Autodesk Fusion 360 part; units mm, degrees
(part 5 of 5)
sketch "Sketch1" plane through (0, 0, 0) normal (0, 0, 1) x (1, 0, 0)
  circle A0 centre (0, 0) radius 1.5
  line L0 (0, 0) -> (29.5, 0) construction
  circle A1 centre (29.5, 0) radius 1.5
  arc A2 (11.3878, -17.4724) -> (12.4, -15.6206) centre (10.2, -15.6206) ccw construction
  line L1 (3, -19.6) -> (3, -7.6) construction
  arc A3 (18.1137, -9.9501) -> (17.1, -11.8029) centre (19.3, -11.8029) ccw construction
  line L2 (29.5, 5) -> (28.4595, 5)
  line L3 (11.9527, 9.1208) -> (3.8379, 5.5832)
  arc A4 (1.2, -13.6) -> (-0.8, -13.6) centre (0.2, -13.6) ccw construction
  arc A5 (13.4019, -3.7339) -> (16.0981, -3.7339) centre (14.75, -1.6285) ccw construction
  arc A6 (33.75, -2.6339) -> (29.5, 5) centre (29.5, 0) ccw
  circle A7 centre (0, 0) radius 1.5
  line L4 (12.4, -11.8029) -> (12.4, -15.6206) construction
  arc A8 (7.2, -16.1338) -> (10.5878, -17.9855) centre (9.4, -16.1338) ccw construction
  arc A9 (17.5473, 9.1208) -> (11.9527, 9.1208) centre (14.75, 2.704) ccw
  line L5 (7.2, -16.1338) -> (7.2, -9.4629) construction
  line L6 (9.0471, -8.4523) -> (11.3863, -9.9501) construction
  arc A10 (-3.8, -4.2143) -> (-4.25, -2.6339) centre (-6.8, -4.2143) ccw construction
  arc A11 (9.3018, 1.2017) -> (9.1273, -0.9969) centre (9.8014, 0.0558) ccw construction
  line L7 (25.6621, 5.5832) -> (17.5473, 9.1208)
  line L8 (1.0405, 5) -> (0, 5)
  line L9 (15.0697, 3.4373) -> (20.1982, 1.2017) construction
  arc A12 (22.3, -9.4629) -> (20.4529, -8.4523) centre (21.1, -9.4629) ccw construction
  arc A13 (1.0405, 5) -> (3.8379, 5.5832) centre (1.0405, 12) ccw
  line L10 (17.1, -15.6206) -> (17.1, -11.8029) construction
  line L11 (9.3018, 1.2017) -> (14.4303, 3.4373) construction
  circle A14 centre (29.5, 0) radius 1.5
  arc A15 (33.75, -2.6339) -> (33.3, -4.2143) centre (36.3, -4.2143) ccw construction
  arc A16 (20.3727, -0.9969) -> (20.1982, 1.2017) centre (19.6986, 0.0558) ccw construction
  arc A17 (0, 5) -> (-4.25, -2.6339) centre (0, 0) ccw
  line L12 (18.9122, -17.9855) -> (18.1122, -17.4724) construction
  line L13 (5, -7.6) -> (5, -19.6) construction
  arc A18 (15.0697, 3.4373) -> (14.4303, 3.4373) centre (14.75, 2.704) ccw construction
  line L14 (11.3878, -17.4724) -> (10.5878, -17.9855) construction
  line L15 (18.1137, -9.9501) -> (20.4529, -8.4523) construction
  arc A19 (12.4, -11.8029) -> (11.3863, -9.9501) centre (10.2, -11.8029) ccw construction
  arc A20 (5, -7.6) -> (3, -7.6) centre (4, -7.6) ccw construction
  line L16 (24.5, -19.6) -> (24.5, -7.6) construction
  arc A21 (25.6621, 5.5832) -> (28.4595, 5) centre (28.4595, 12) ccw
  line L17 (20.3727, -0.9969) -> (16.0981, -3.7339) construction
  arc A22 (3, -19.6) -> (5, -19.6) centre (4, -19.6) ccw construction
  arc A23 (18.9122, -17.9855) -> (22.3, -16.1338) centre (20.1, -16.1338) ccw construction
  arc A24 (17.1, -15.6206) -> (18.1122, -17.4724) centre (19.3, -15.6206) ccw construction
  line L18 (13.4019, -3.7339) -> (9.1273, -0.9969) construction
  arc A25 (9.0471, -8.4523) -> (7.2, -9.4629) centre (8.4, -9.4629) ccw construction
  line L19 (26.5, -7.6) -> (26.5, -19.6) construction
  arc A26 (26.5, -7.6) -> (24.5, -7.6) centre (25.5, -7.6) ccw construction
  line L20 (22.3, -9.4629) -> (22.3, -16.1338) construction
  arc A27 (30.3, -13.6) -> (28.3, -13.6) centre (29.3, -13.6) ccw construction
  circle A28 centre (0, 0) radius 5
  circle A29 centre (29.5, 0) radius 5
  line L21 (23.2644, 0.0831) -> (15.1496, 3.6207)
  arc A30 (15.1496, 3.6207) -> (14.3504, 3.6207) centre (14.75, 2.704) ccw
  line L22 (14.3504, 3.6207) -> (6.2356, 0.0831)
  line L23 (6.2356, 0.0831) -> (4.9783, -0.4649)
  line L24 (23.2644, 0.0831) -> (24.5217, -0.4649)
  point P0 (14.75, -5.1)
  dimension "d35" = 3
  dimension "d36" = 29.5
  dimension "d37" = 3
  dimension "d38" = -6
  constraint coincident A0.centre L0.start
  constraint horizontal L0
  constraint coincident L0.end A1.centre
  constraint concentric A7 A28
  constraint coincident A10.end A28
  constraint coincident A6.start A29
  constraint tangent A15 A29
  constraint coincident A28 L23.end
  constraint collinear L22 L23
  constraint coincident A29 L24.end
  constraint collinear L21 L24
  measures "d35" diameter of A0
  measures "d36" distance of A0.centre L0.end
  measures "d37" diameter of A1
extrude "Extrude3" add sketch "Sketch1" along normal blind 2
fillet "Fillet3" radius 3 2 edges at (4.9783, -0.4649, 1) (24.5217, -0.4649, 1)

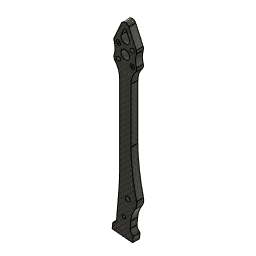
design "arm_front_6mm"
Autodesk Fusion 360 part; units mm, degrees
sketch "Sketch1" plane through (0, 0, 0) normal (0, 0, 1) x (1, 0, 0)
  circle A0 centre (0, 0) radius 3.8
  dimension "d2" = 7.6
  constraint coincident A0.centre origin
  measures "d2" diameter of A0
sketch "Sketch2" plane through (0, 0, 0) normal (0, 0, 1) x (1, 0, 0)
  arc A0 (28.2898, -146.7842) -> (30.0064, -147.0869) centre (30.8779, -137.1249) ccw construction
  arc A1 (9.3424, -112.1265) -> (12.7274, -116.0513) centre (22.2229, -104.4394) ccw construction
  line L0 (9.8518, -167.6702) -> (17.4021, -163.8233) construction
  circle A2 centre (2.1789, -108.5649) radius 3.375 construction
  line L1 (100.4519, -39.9064) -> (12.7274, -116.0513) construction
  line L2 (28.2898, -146.7842) -> (23.615, -145.5316) construction
  arc A3 (30.9564, -136.2283) -> (29.2133, -136.2283) centre (30.0848, -146.1903) ccw construction
  arc A4 (2.3786, -152.7505) -> (5.279, -154.7068) centre (4.371, -152.9248) ccw construction
  arc A5 (100.4519, -39.9064) -> (105.7604, -37.9868) centre (99.4908, -28.9484) ccw construction
  line L3 (18.4399, -134.3914) -> (17.361, -146.7224) construction
  line L4 (22.8776, -144.4785) -> (23.4829, -137.5592) construction
  arc A6 (-11.1082, -168.6356) -> (3.7484, -173.4033) centre (-3.1387, -169.3329) ccw construction
  arc A7 (23.3547, -162.6662) -> (17.4021, -163.8233) centre (22.396, -173.6243) ccw construction
  line L5 (-5.7907, -107.8678) -> (-7.6374, -128.9799)
  arc A8 (-9.2616, -147.5287) -> (-11.8245, -142.975) centre (-13.8718, -147.1253) ccw construction
  line L6 (4.7746, -145.5276) -> (6.1209, -144.398) construction
  line L7 (24.392, -136.6501) -> (29.2133, -136.2283) construction
  arc A9 (-10.9528, -133.0126) -> (-7.6374, -128.9799) centre (-12.2491, -128.5675) ccw
  circle A10 centre (27.1493, -126.0578) radius 1.5 construction
  line L8 (6.9668, -134.7286) -> (5.8373, -133.3824) construction
  line L9 (-9.2616, -147.5287) -> (-11.1082, -168.6356) construction
  arc A11 (22.8776, -144.4785) -> (23.615, -145.5316) centre (23.8738, -144.5656) ccw construction
  circle A12 centre (24.4911, -156.4418) radius 1.5 construction
  arc A13 (7.9279, -124.4303) -> (4.7319, -125.8533) centre (6.7243, -126.0276) ccw construction
  arc A14 (9.8518, -167.6702) -> (3.7484, -173.4033) centre (16.6616, -181.0354) ccw construction
  circle A15 centre (-3.7013, -153.9753) radius 1.5 construction
  arc A16 (9.3424, -112.1265) -> (-5.7907, -107.8678) centre (2.1789, -108.5649) ccw construction
  arc A17 (24.392, -136.6501) -> (23.4829, -137.5592) centre (24.4791, -137.6463) ccw construction
  line L10 (15.7692, -149.4168) -> (5.279, -154.7068) construction
  line L11 (2.3786, -152.7505) -> (2.6542, -149.601) construction
  circle A18 centre (31.9218, -131.7454) radius 1.5 construction
  line L12 (7.9279, -124.4303) -> (17.3401, -131.4615) construction
  circle A19 centre (-3.1387, -169.3329) radius 3.375 construction
  line L13 (4.4564, -129.0028) -> (4.7319, -125.8533) construction
  arc A20 (4.4564, -129.0028) -> (5.8373, -133.3824) centre (10.4336, -129.5257) ccw construction
  circle A21 centre (-1.043, -123.5913) radius 1.5
  spline S0 degree 5 poles (17.3401, -131.4615) (17.4524, -131.5454) (17.6596, -131.7229) (17.9183, -132.0182) (18.171, -132.4622) (18.3701, -133.0729) (18.4504, -133.5889) (18.4644, -133.9863) (18.4517, -134.2556) (18.4399, -134.3914) knots 0 0 0 0 0 0 0.2 0.4 0.6 0.8 1 1 1 1 1 1 construction
  circle A22 centre (30.1786, -151.6693) radius 1.5 construction
  spline S1 degree 5 poles (17.361, -146.7224) (17.3492, -146.8581) (17.3149, -147.1256) (17.232, -147.5145) (17.0634, -148.0088) (16.7613, -148.5756) (16.4353, -148.9689) (16.1293, -149.2149) (15.8944, -149.3537) (15.7692, -149.4168) knots -1 -1 -1 -1 -1 -1 -0.8 -0.6 -0.4 -0.2 0 0 0 0 0 0 construction
  arc A23 (4.7746, -145.5276) -> (2.6542, -149.601) centre (8.6313, -150.1239) ccw construction
  line L14 (-10.9528, -133.0126) -> (-11.8245, -142.975)
  line L15 (6.1209, -144.398) -> (6.9668, -134.7286) construction
  circle A24 centre (2.1789, -108.5649) radius 2
  line L16 (0.1865, -108.3907) -> (-1.6602, -129.5027) construction
  arc A25 (4.317, -130.0255) -> (6.882, -134.5726) centre (8.9303, -130.4201) ccw
  line L17 (6.882, -134.5726) -> (6.0108, -144.535)
  line L18 (-11.3887, -137.9938) -> (6.5439, -139.5619)
  circle A26 centre (2.1789, -108.5649) radius 8
  line L19 (4.317, -130.0255) -> (4.8399, -124.0484)
  spline S2 degree 5 poles (4.8399, -124.0484) (4.8815, -123.5731) (4.9918, -122.6298) (5.2386, -121.2367) (5.7136, -119.4197) (6.5081, -117.2134) (7.2997, -115.51) (7.9954, -114.2779) (8.5094, -113.4794) (8.779, -113.0859) knots 0 0 0 0 0 0 0.2 0.4 0.6 0.8 1 1 1 1 1 1
  line L20 (0, 0) -> (13.2638, -13.2638) construction
  line L21 (0, 0) -> (18.7579, 0) construction
  line L22 (7.566, -5.4447) -> (6.7175, -4.5962)
  arc A27 (6.7175, -4.5962) -> (4.5962, -6.7175) centre (5.6569, -5.6569) ccw
  line L23 (4.5962, -6.7175) -> (5.4447, -7.566)
  arc A28 (5.4447, -7.566) -> (7.566, -5.4447) centre (6.5054, -6.5054) ccw
  line L24 (7.566, -7.566) -> (4.5962, -4.5962) construction
  arc A29 (4.5962, 6.7175) -> (6.7175, 4.5962) centre (5.6569, 5.6569) ccw
  line L25 (5.4447, 7.566) -> (4.5962, 6.7175)
  arc A30 (7.566, 5.4447) -> (5.4447, 7.566) centre (6.5054, 6.5054) ccw
  line L26 (6.7175, 4.5962) -> (7.566, 5.4447)
  arc A31 (-6.7175, 4.5962) -> (-4.5962, 6.7175) centre (-5.6569, 5.6569) ccw
  line L27 (-7.566, 5.4447) -> (-6.7175, 4.5962)
  arc A32 (-5.4447, 7.566) -> (-7.566, 5.4447) centre (-6.5054, 6.5054) ccw
  line L28 (-4.5962, 6.7175) -> (-5.4447, 7.566)
  arc A33 (-4.5962, -6.7175) -> (-6.7175, -4.5962) centre (-5.6569, -5.6569) ccw
  line L29 (-5.4447, -7.566) -> (-4.5962, -6.7175)
  arc A34 (-7.566, -5.4447) -> (-5.4447, -7.566) centre (-6.5054, -6.5054) ccw
  line L30 (-6.7175, -4.5962) -> (-7.566, -5.4447)
  line L31 (0, 0) -> (0, -132.816) construction
  line L32 (-5, -105.0346) -> (-5, -20)
  spline S3 degree 5 poles (-5.7907, -107.8678) (-5.7382, -107.2682) (-5.6366, -106.0687) (-5.4939, -104.2686) (-5.3227, -101.867) (-5.1465, -98.863) (-5.0482, -96.458) (-5.0088, -94.6529) (-5, -93.4489) (-5, -92.8467) knots 0 0 0 0 0 0 0.2 0.4 0.6 0.8 1 1 1 1 1 1
  line L33 (5, -101.0789) -> (5, -20)
  line L34 (0, 24.5) -> (0, 0) construction
  circle A35 centre (0, 21) radius 3.5
  circle A36 centre (-6.5054, 6.5054) radius 3.5
  circle A37 centre (-6.5054, -6.5054) radius 3.5
  line L35 (0, 0) -> (-9, 0) construction
  arc A38 (-9.8421, -5.4488) -> (-9.8421, 5.4488) centre (-27.0494, 0) ccw
  line L36 (-5, -20) -> (5, -20) construction
  arc A39 (-5, -20) -> (-9.1588, -8.7878) centre (-22.1936, -20) ccw
  line L37 (-9.6985, 7.9385) -> (-3.1931, 22.4331)
  line L38 (9.6985, 7.9385) -> (3.1931, 22.4331)
  circle A40 centre (6.5054, 6.5054) radius 3.5
  arc A41 (9.8421, 5.4488) -> (9.8421, -5.4488) centre (27.0494, 0) ccw
  arc A42 (9.1588, -8.7878) -> (5, -20) centre (22.1936, -20) ccw
  circle A43 centre (6.5054, -6.5054) radius 3.5
  circle A44 centre (0, 0) radius 3.8
  circle A45 centre (0, 12) radius 3.75
  line L39 (0.9091, 19.0167) -> (3.409, 13.5625)
  line L40 (-0.9091, 19.0167) -> (-3.409, 13.5625)
  arc A46 (0.9091, 19.0167) -> (-0.9091, 19.0167) centre (0, 18.6) ccw
  spline S4 degree 5 poles (9.9567, -106.6925) (9.5878, -105.1601) (8.8852, -102.0894) (7.9369, -97.465) (6.8666, -91.2667) (5.829, -83.4768) (5.2712, -77.2155) (5.0493, -72.5017) (5, -69.3506) (5, -67.773) knots 0 0 0 0 0 0 0.2 0.4 0.6 0.8 1 1 1 1 1 1
  point P0 (6.5439, -139.5619)
  point P1 (0, 24.5)
  dimension "d3" = 4
  dimension "d4" = -6
  dimension "d5" = 6
  dimension "d6" = 45
  dimension "d8" = 3
  dimension "d9" = 6.5
  dimension "d12" = 4.2
  dimension "d14" = 360
  dimension "d16" = 5
  dimension "d17" = 5
  dimension "d18" = 7
  dimension "d19" = 24.5
  dimension "d20" = 7
  dimension "d21" = 7
  dimension "d22" = 9
  dimension "d23" = 20
  dimension "d24" = 7.5
  dimension "d26" = 12
  dimension "d27" = 1
  constraint concentric A2 A24
  constraint symmetric A8.end L16 L17.end
  constraint symmetric A9.start L16 A25.end
  constraint symmetric L5.end L16 A25.start
  constraint symmetric A9 L16 A25
  constraint midpoint L14 L18.start
  constraint coincident P0 L18.end
  constraint perpendicular L17 L18
  constraint concentric A24 A26
  constraint coincident L5.start A26
  constraint tangent L5 A26
  constraint parallel L13 L19
  constraint coincident A26 S2.end
  constraint tangent A26 S2
  constraint horizontal L21
  constraint coincident L20.start L21.start
  constraint tangent L22 A27
  constraint tangent A27 L23
  constraint parallel L22 L23
  constraint tangent L23 A28
  constraint tangent L22 A28
  constraint midpoint A28 L24.start
  constraint midpoint A27 L24.end
  constraint coincident L20 L24.end
  constraint parallel L20 L24
  constraint perpendicular L21 L31
  constraint coincident A16 L32.start
  constraint parallel L31 L32
  constraint coincident L32 S3.end
  constraint coincident A16 L33.start
  constraint parallel L31 L33
  constraint coincident P1 L34.start
  constraint perpendicular L21 L34
  constraint coincident P1 A35
  constraint concentric A32 A36
  constraint concentric A34 A37
  constraint perpendicular L34 L35
  constraint coincident L35.end A38
  constraint coincident A36 A38.end
  constraint coincident A37 A38.start
  constraint tangent A36 A38
  constraint tangent A37 A38
  constraint horizontal L36
  constraint tangent A37 A39
  constraint coincident A37 A39.end
  constraint tangent L32 A39
  constraint coincident L34 A35.centre
  constraint coincident A36 L37.start
  constraint coincident A35 L37.end
  constraint tangent A35 L37
  constraint tangent A36 L37
  constraint symmetric L32.end L34 L33.end
  constraint symmetric L34 A36 A40
  constraint symmetric L34 A38.start A41.end
  constraint symmetric L34 A38.end A41.start
  constraint symmetric L34 A38 A41
  constraint symmetric L34 A39.end A42.start
  constraint symmetric L34 A39 A42
  constraint symmetric L34 L37.start L38.start
  constraint symmetric L34 L37.end L38.end
  constraint symmetric L34 A37 A43
  constraint coincident L34 A45.centre
  constraint coincident A45 L39.end
  constraint tangent A45 L39
  constraint coincident A45 L40.end
  constraint tangent A45 L40
  constraint tangent L39 A46
  constraint tangent L40 A46
  constraint coincident A26 S4.start
  constraint coincident L33 S4.end
  constraint tangent A26 S4
  measures "d3" diameter of A24
  measures "d5" distance of A25.start L19.end
  measures "d6" angle of L20 L21
  measures "d8" diameter of A27
  measures "d9" distance of L24.end L20.start
  measures "d12" distance of L24.start L24.end
  measures "d16" distance of L31 L32
  measures "d17" distance of L31 L33
  measures "d18" diameter of A35
  measures "d19" distance of L20.start P1
  measures "d20" diameter of A36
  measures "d21" diameter of A37
  measures "d22" distance of L20.start L35.end
  measures "d23" distance of L20.start L36
  measures "d24" diameter of A45
  measures "d26" distance of L20.start A45.centre
  measures "d27" radius of A46
extrude "Extrude1" add sketch "Sketch2" along normal blind 6 contours L5 A9 L14 A25 L17 L18 A26 L19 S2 | A26 L32 S3 | A26 | A26 L32 L33 A35 A36 A37 A38 A39 L37 L38 A40 A41 A42 A43 A45 L39 L40 | A26 L33 S4 | A37 | A43 | A36 | A40 | A35 L39 L40 A46 picked at (0.167, 22.8547)
equation "d9 = ( ( 7.6 / 2 ) * 1 mm ) + 2.7 mm"

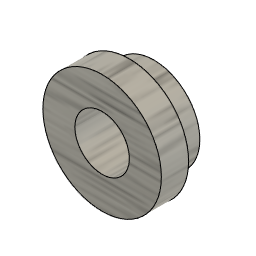
design "nut"
Autodesk Fusion 360 part; units mm, degrees
sketch "Sketch1" plane through (0, 0, 0) normal (0, 0, 1) x (1, 0, 0)
  circle A0 centre (0, 0) radius 4.35
  circle A1 centre (0, 0) radius 2
  dimension "d1" = 8.7
  dimension "d2" = 4
  constraint coincident A0.centre A1.centre
  measures "d1" diameter of A0
  measures "d2" diameter of A1
extrude "Extrude1" add sketch "Sketch1" along normal blind 2
sketch "Sketch2" plane through (0, 0, 0) normal (0, 0, -1) x (-1, 0, 0)
  circle A0 centre (0, 0) radius 2
  circle A1 centre (0, 0) radius 4.35
  circle A2 centre (0, 0) radius 2
  circle A3 centre (0, 0) radius 3.375
  dimension "d5" = 6.75
  constraint concentric A2 A3
  measures "d5" diameter of A3
extrude "Extrude2" add sketch "Sketch2" along normal blind 1.8 contours A3
